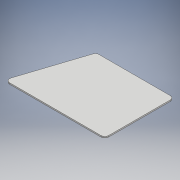
# Autodesk Inventor part: VentanaLateralDelantera
Saved by Autodesk Inventor 2017 (Build 210142000, 142)
## iProperties
Part Number: VentanaLateralDelantera
Material: Genérico
Document SubType Name: Modeling
Designer: Ghost
Density: 1 g/cm^3
Appearance: Valor por defecto
Author: Ghost
Autodesk Inventor part; units mm, degrees
ref_plane "YZ Plane" through (0, 0, 0) normal (1, 0, 0) x (0, 1, 0)
ref_plane "XZ Plane" through (0, 0, 0) normal (0, 1, 0) x (-1, 0, 0)
ref_plane "XY Plane" through (0, 0, 0) normal (0, 0, 1) x (1, 0, 0)
sketch "Boceto1" plane through (0, 0, 0) normal (0, 0, 1) x (1, 0, 0)
  line L0 (0.8523, 2.6189) -> (11.8523, 36.4189)
  line L1 (13.7541, 37.8) -> (52.7541, 37.8)
  line L2 (54.7541, 35.8) -> (54.7541, 2)
  line L3 (52.7541, 0) -> (2.7541, 0)
  arc A0 (13.7541, 37.8) -> (11.8523, 36.4189) centre (13.7541, 35.8) ccw
  arc A1 (54.7541, 35.8) -> (52.7541, 37.8) centre (52.7541, 35.8) ccw
  arc A2 (52.7541, 0) -> (54.7541, 2) centre (52.7541, 2) ccw
  arc A3 (0.8523, 2.6189) -> (2.7541, 0) centre (2.7541, 2) ccw
  point P0 (0, 0)
  point P1 (12.3018, 37.8)
  point P2 (54.7541, 37.8)
  point P3 (54.7541, 0)
  dimension "d3" = 2
  dimension "d6" = 33.8
  dimension "d7" = 39
  dimension "d8" = 50
  constraints: 8 end point, 8 point on circle, 8 point on line, 8 tangent, 4 centre point, 3 equal radius, 2 perpendicular, 1 horizontal
  measures "d3" radius of A0
  measures "d6" distance of A2.centre A1.centre
  measures "d7" distance of A1.centre A0.centre
  measures "d8" distance of A2.centre A3.centre
extrude "Extrusión1" add sketch "Boceto1" along normal blind 0.75
